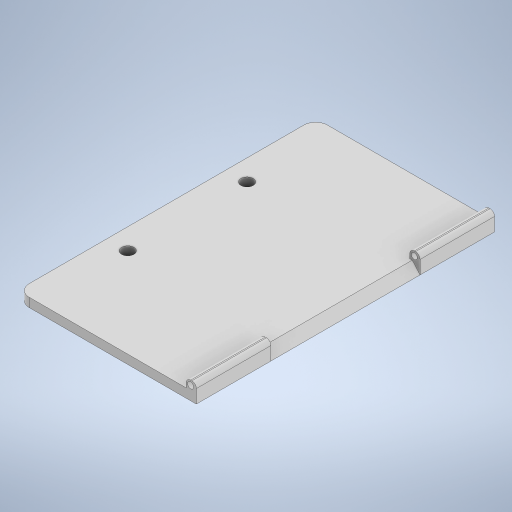
# Autodesk Inventor part: Cover
Saved by Autodesk Inventor 2023 (Build 270158000, 158)
## iProperties
Created: 2023-03-07
Part Number: Cover
Material: Типовые
Document SubType Name: Modeling
Designer: Josh
Density: 1 g/cm^3
Appearance: По умолчанию
Author: Josh
Autodesk Inventor part; units mm, degrees
ref_plane "YZ Plane" through (0, 0, 0) normal (1, 0, 0) x (0, 1, 0)
ref_plane "XZ Plane" through (0, 0, 0) normal (0, 1, 0) x (-1, 0, 0)
ref_plane "XY Plane" through (0, 0, 0) normal (0, 0, 1) x (1, 0, 0)
sketch "Эскиз2" plane through (0, 0, 0) normal (0, 0, 1) x (1, 0, 0)
  line L0 (0, 0) -> (60, 0)
  line L1 (60, 0) -> (60, 3)
  line L2 (60, 3) -> (0, 3)
  line L3 (0, 3) -> (0, 0)
  dimension "d14" = 60
  dimension "d15" = 3
  constraints: 8 end point, 2 parallel, 1 horizontal, 1 perpendicular
  measures "d14" distance between parallel lines of L3 L1
  measures "d15" distance between parallel lines of L0 L2
extrude "Выдавливание2" add sketch "Эскиз2" along normal mid plane 100
sketch "Эскиз4" plane through (0, 3, 50) normal (0, 1, 0) x (1, 0, 0)
  circle A0 centre (7, 30) radius 2.05
  line L0 (0, 50) -> (60, 50)
  line L1 (60, 100) -> (60, 0) projected
  circle A1 centre (7, 70) radius 2.05
  dimension "d19" = 4.1
  dimension "d20" = 53
  dimension "d21" = 40
  constraints: 2 centre point, 2 end point, 1 horizontal, 1 midpoint, 1 symmetric about line, 1 other
  measures "d19" diameter of A0
  measures "d20" distance from line of L1 A0.centre
  measures "d21" distance of A1.centre A0.centre
extrude "Выдавливание3" cut sketch "Эскиз4" against normal through all
fillet "Сопряжение1" radius 4 2 edges at (0, 1.5, 50) (0, 1.5, -50)
sketch "Эскиз5" plane through (60, 3, 50) normal (0, 1, 0) x (1, 0, 0)
  line L0 (0, 100) -> (0, 0) projected
  line L1 (0, 0) -> (-56, 0) projected
  line L2 (0, 100) -> (-3.42, 100)
  line L3 (-3.42, 100) -> (-3.42, 0)
  line L4 (-3.42, 0) -> (0, 0)
  line L5 (0, 0) -> (0, 100)
  point P0 (-60, 50)
  dimension "d25" = 3.42
  constraints: 8 end point, 2 parallel, 1 horizontal, 1 perpendicular, 1 point on line
  measures "d25" distance between parallel lines of L0 L3
extrude "Выдавливание4" add sketch "Эскиз5" along normal blind 3
sketch "Эскиз6" plane through (0, 0, 50) normal (0, 0, 1) x (1, 0, 0)
  circle A0 centre (58.08, 4.5) radius 1
  line L0 (56.58, 6) -> (60, 6) projected
  line L1 (56.58, 3) -> (56.58, 6) projected
  point P0 (0, 0)
  dimension "d28" = 2
  dimension "d29" = 1.5
  dimension "d30" = 1.5
  constraints: 1 centre point
  measures "d28" diameter of A0
  measures "d29" distance from line of A0.centre L0
  measures "d30" distance from line of L1 A0.centre
extrude "Выдавливание5" cut sketch "Эскиз6" against normal through all
sketch "Эскиз7" plane through (60, 6, 50) normal (0, 1, 0) x (1, 0, 0)
  line L0 (-3.42, 100) -> (-3.42, 0) projected
  line L1 (0, 0) -> (0, 100) projected
  line L2 (-3.42, 25) -> (0, 25)
  line L3 (0, 25) -> (0, 75)
  line L4 (0, 75) -> (-3.42, 75)
  line L5 (-3.42, 75) -> (-3.42, 25)
  line L6 (-3.42, 0) -> (-56, 0) projected
  point P0 (-60, 50)
  point P1 (-3.42, 75)
  point P2 (0, 25)
  dimension "d33" = 50
  dimension "d34" = 25
  constraints: 8 end point, 2 parallel, 2 point on line, 1 horizontal, 1 perpendicular
  measures "d33" distance between parallel lines of L2 L4
  measures "d34" distance between parallel lines of L6 L2
extrude "Выдавливание6" cut sketch "Эскиз7" against normal blind 3
fillet "Сопряжение2" radius 1.5 4 edges at (60, 6, 37.5) (56.58, 6, 37.5) (60, 6, -37.5) (56.58, 6, -37.5)
sketch "Эскиз8" plane through (56.58, 3, -25) normal (0, 0, 1) x (1, 0, 0)
  line L0 (3.42, -3) -> (3.42, 1.5) projected
  line L1 (0, 0.9343) -> (3.42, -3)
  line L2 (3.42, -3) -> (-52.58, -3) projected
  line L3 (0, 0) -> (0, 1.5) projected
  line L4 (0, 0.9343) -> (3.42, 0.9343)
  point P0 (-56.58, -3)
  dimension "d38" = 49
  constraints: 4 end point, 2 point on line, 1 perpendicular
  measures "d38" angle of L2 L1
extrude "Выдавливание7" cut sketch "Эскиз8" along normal up to surface (50 mm away)
